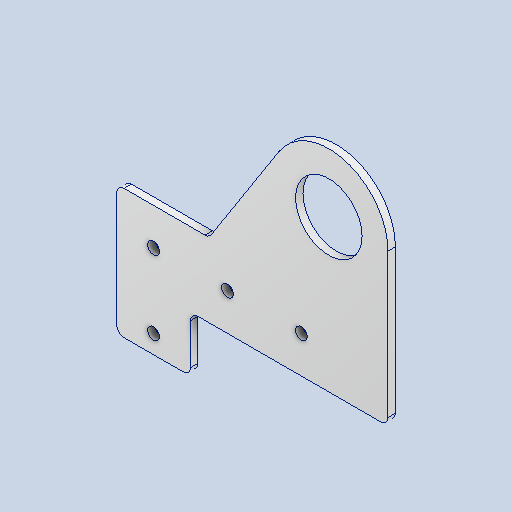
# Autodesk Inventor part: dribl-v3-Plate-1
Saved by Autodesk Inventor 2025.2 (Build 292293000, 293)
## iProperties
Created: 2025-04-04
Part Number: dribl-v3-Plate-1
Material: アルミニウム 6061
Document SubType Name: Modeling
Designer: haruy
Density: 2.7 g/cm^3
Appearance: アルミニウム - フラット
Author: haruy
Autodesk Inventor part; units mm, degrees
ref_plane "YZ Plane" through (0, 0, 0) normal (1, 0, 0) x (0, 1, 0)
ref_plane "XZ Plane" through (0, 0, 0) normal (0, 1, 0) x (-1, 0, 0)
ref_plane "XY Plane" through (0, 0, 0) normal (0, 0, 1) x (1, 0, 0)
derived "dribl-v3-Sketch-Base.ipt"
sketch "スケッチ5" plane through (-180, -184.3334, -303) normal (0, 0, 1) x (1, 0, 0)
  circle A0 centre (37.42, 41) radius 16 projected
  line L0 (0, -248) -> (0, 1189.5) projected
  line L1 (560, 20) -> (0, 20) projected
  circle A1 centre (10, 10) radius 1.6 projected
  circle A2 centre (30, 10) radius 1.6 projected
  line L2 (0, 0) -> (560, 0) projected
  line L3 (280, 20) -> (280, 0) projected
  circle A3 centre (522.58, 41) radius 16 projected
  circle A4 centre (530, 10) radius 1.6 projected
  circle A5 centre (550, 10) radius 1.6 projected
  circle A6 centre (-10, 10) radius 1.6 projected
  circle A7 centre (-10, -10) radius 1.6 projected
  line L4 (-20, 1189.5) -> (-20, -248) projected
  circle A8 centre (570, 10) radius 1.6 projected
  circle A9 centre (570, -10) radius 1.6 projected
  circle A10 centre (37.42, 41) radius 16
  circle A11 centre (37.42, 41) radius 9
  line L5 (0, 20) -> (5, 20)
  line L6 (5, 20) -> (5, 63.0652)
  line L7 (5, 63.0652) -> (0, 63.0652)
  line L8 (0, 63.0652) -> (0, 20)
  line L9 (23.9403, 49.6196) -> (5, 20)
  line L10 (0, 20) -> (-20, 20)
  line L11 (-20, -15) -> (0, -15)
  line L12 (53.42, 41) -> (53.42, 0)
  line L13 (420, 0) -> (420, 20) projected
  line L14 (560, -248) -> (560, 1189.5) projected
  line L15 (415, 20) -> (415, 0) projected
  circle A12 centre (404.9, 46) radius 16 projected
  circle A13 centre (404.9, 46) radius 5.1 projected
  line L16 (404.9, 46) -> (404.9, 0) projected
  line L17 (394.8, 20) -> (394.8, 0) projected
  circle A14 centre (404.9, 66) radius 5.1 projected
  circle A15 centre (404.9, 66) radius 10.1 projected
  line L18 (394.8, 20) -> (394.8, 66) projected
  line L19 (415, 20) -> (415, 66) projected
  line L20 (394.8, 66) -> (415, 66) projected
  line L21 (415, 66) -> (415, 76.1) projected
  line L22 (415, 76.1) -> (394.8, 76.1) projected
  line L23 (394.8, 76.1) -> (394.8, 66) projected
  line L24 (399.8, 46) -> (399.8, 66) projected
  line L25 (410, 66) -> (410, 46) projected
  circle A16 centre (410, 10) radius 1.6 projected
  circle A17 centre (400, 10) radius 1.6 projected
  line L26 (394.8, 0) -> (415, 0) projected
  line L27 (415, 0) -> (415, 20) projected
  line L28 (415, 20) -> (394.8, 20) projected
  line L29 (394.8, 20) -> (394.8, 0) projected
  circle A18 centre (404.9, 41) radius 5.1 projected
  line L30 (399.8, 46) -> (399.8, 41) projected
  line L31 (410, 46) -> (410, 41) projected
  circle A19 centre (371.4, 45) radius 11 projected
  circle A20 centre (371.4, 45) radius 2 projected
  circle A21 centre (37.42, 41) radius 12.5 projected
  circle A22 centre (522.58, 41) radius 12.5 projected
  line L32 (522.58, 53.5) -> (37.42, 53.5) projected
  line L33 (37.42, 28.5) -> (522.58, 28.5) projected
  line L34 (360.4, 45) -> (360.4, 0) projected
  line L35 (382.4, 45) -> (382.4, 0) projected
  circle A23 centre (366.4, 10) radius 1.5 projected
  circle A24 centre (376.4, 10) radius 1.5 projected
  line L36 (449.4, 45) -> (449.4, 0) projected
  line L37 (427.4, 45) -> (427.4, 0) projected
  circle A25 centre (438.4, 45) radius 11 projected
  circle A26 centre (438.4, 45) radius 2 projected
  circle A27 centre (443.4, 10) radius 1.5 projected
  circle A28 centre (433.4, 10) radius 1.5 projected
  point P0 (180, 184.3334)
  point P1 (53.42, 41)
  point P2 (23.9403, 49.6196)
  dimension "d1" = 32
  dimension "d2" = 18
  dimension "d3" = 5
  dimension "d4" = 5
  constraints: 16 end point, 4 perpendicular, 4 point on line, 2 centre point, 2 coincident, 2 parallel, 2 point on circle, 2 tangent, 1 horizontal
  measures "d1" diameter of A10
  measures "d2" diameter of A11
  measures "d3" distance of L7.end L6.end
  measures "d4" distance from line of L11 A7.centre
extrude "押し出し1" add sketch "スケッチ5" against normal blind 2 contours A0 L33 A21 L32 | L12 L33 A0 | L32 A21 L33 A0 | L33 L12 L1 L9 A0 | A21 | L12 L2 L0 L1 | L0 L11 L4 L10
fillet "フィレット1" radius 2 6 edges at (-126.58, -184.3334, -304) (-180, -184.3334, -304) (-180, -199.3334, -304) (-200, -199.3334, -304) (-200, -164.3334, -304) (-175, -164.3334, -304)
